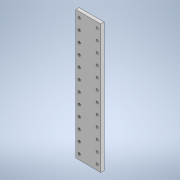
# Autodesk Inventor part: Base_plate
Saved by Autodesk Inventor 2022 (Build 260153000, 153)
## iProperties
Created: 2022-01-26
Part Number: Base_plate
Material: Generic
Document SubType Name: Modeling
Designer: Emazuddin Alif
Density: 1 g/cm^3
Appearance: Default
Author: Emazuddin Alif
Autodesk Inventor part; units mm, degrees
ref_plane "YZ Plane" through (0, 0, 0) normal (1, 0, 0) x (0, 1, 0)
ref_plane "XZ Plane" through (0, 0, 0) normal (0, 1, 0) x (-1, 0, 0)
ref_plane "XY Plane" through (0, 0, 0) normal (0, 0, 1) x (1, 0, 0)
sketch "Sketch1" plane through (0, 0, 0) normal (0, 0, 1) x (1, 0, 0)
  line L0 (44.45, -228.6) -> (-44.45, -228.6)
  line L1 (-44.45, -228.6) -> (-44.45, 228.6)
  line L2 (-44.45, 228.6) -> (44.45, 228.6)
  line L3 (44.45, 228.6) -> (44.45, -228.6)
  line L4 (44.45, -228.6) -> (-44.45, 228.6) construction
  line L5 (-44.45, -228.6) -> (44.45, 228.6) construction
  line L6 (0, 60.7039) -> (0, -84.4127)
  circle A0 centre (-31.75, -209.55) radius 3.9688
  circle A1 centre (31.75, -209.55) radius 3.9688
  circle A2 centre (-31.75, -171.45) radius 3.9688
  circle A3 centre (31.75, -171.45) radius 3.9688
  circle A4 centre (-31.75, -133.35) radius 3.9688
  circle A5 centre (31.75, -133.35) radius 3.9688
  circle A6 centre (-31.75, -95.25) radius 3.9688
  circle A7 centre (31.75, -95.25) radius 3.9688
  circle A8 centre (-31.75, -57.15) radius 3.9688
  circle A9 centre (31.75, -57.15) radius 3.9688
  circle A10 centre (-31.75, -19.05) radius 3.9688
  circle A11 centre (31.75, -19.05) radius 3.9688
  circle A12 centre (-31.75, 19.05) radius 3.9688
  circle A13 centre (31.75, 19.05) radius 3.9688
  circle A14 centre (-31.75, 57.15) radius 3.9688
  circle A15 centre (31.75, 57.15) radius 3.9688
  circle A16 centre (-31.75, 95.25) radius 3.9688
  circle A17 centre (31.75, 95.25) radius 3.9688
  circle A18 centre (-31.75, 133.35) radius 3.9688
  circle A19 centre (31.75, 133.35) radius 3.9688
  circle A20 centre (-31.75, 171.45) radius 3.9688
  circle A21 centre (31.75, 171.45) radius 3.9688
  circle A22 centre (-31.75, 209.55) radius 3.9688
  circle A23 centre (31.75, 209.55) radius 3.9688
  point P0 (0, 0)
  dimension "d0" = 457.2
  dimension "d1" = 88.9
  dimension "d2" = 7.9375
  dimension "d3" = 19.05
  dimension "d4" = 12.7
  dimension "d5" = 12.7
  dimension "d8" = 38.1
  constraints: 24 centre point, 14 end point, 2 midpoint, 2 parallel, 2 vertical, 1 horizontal, 1 perpendicular, 1 symmetric about line, 45 other
  measures "d0" distance of L0.end L1.end
  measures "d1" distance of L1.end L2.end
  measures "d2" diameter of A0
  measures "d3" distance from line of L0 A0.centre
  measures "d4" distance from line of L1 A0.centre
  measures "d5" distance from line of L3 A1.centre
  measures "d8" distance of A0.centre A2.centre
extrude "Extrusion1" add sketch "Sketch1" along normal blind 12.192
thread "Thread13" size "5/16-18 UNC" class "2B" standard "ANSI Unified Screw Threads" full length
thread "Thread14" size "5/16-18 UNC" class "2B" standard "ANSI Unified Screw Threads" full length
thread "Thread15" size "5/16-18 UNC" class "2B" standard "ANSI Unified Screw Threads" full length
thread "Thread16" size "5/16-18 UNC" class "2B" standard "ANSI Unified Screw Threads" full length
thread "Thread17" size "5/16-18 UNC" class "2B" standard "ANSI Unified Screw Threads" full length
thread "Thread18" size "5/16-18 UNC" class "2B" standard "ANSI Unified Screw Threads" full length
thread "Thread19" size "5/16-18 UNC" class "2B" standard "ANSI Unified Screw Threads" full length
thread "Thread20" size "5/16-18 UNC" class "2B" standard "ANSI Unified Screw Threads" full length
thread "Thread21" size "5/16-18 UNC" class "2B" standard "ANSI Unified Screw Threads" full length
thread "Thread22" size "5/16-18 UNC" class "2B" standard "ANSI Unified Screw Threads" full length
thread "Thread23" size "5/16-18 UNC" class "2B" standard "ANSI Unified Screw Threads" full length
thread "Thread24" size "5/16-18 UNC" class "2B" standard "ANSI Unified Screw Threads" full length
thread "Thread25" size "5/16-18 UNC" class "2B" standard "ANSI Unified Screw Threads" full length
thread "Thread26" size "5/16-18 UNC" class "2B" standard "ANSI Unified Screw Threads" full length
thread "Thread27" size "5/16-18 UNC" class "2B" standard "ANSI Unified Screw Threads" full length
thread "Thread28" size "5/16-18 UNC" class "2B" standard "ANSI Unified Screw Threads" full length
thread "Thread29" size "5/16-18 UNC" class "2B" standard "ANSI Unified Screw Threads" full length
thread "Thread30" size "5/16-18 UNC" class "2B" standard "ANSI Unified Screw Threads" full length
thread "Thread31" size "5/16-18 UNC" class "2B" standard "ANSI Unified Screw Threads" full length
thread "Thread32" size "5/16-18 UNC" class "2B" standard "ANSI Unified Screw Threads" full length
thread "Thread33" size "5/16-18 UNC" class "2B" standard "ANSI Unified Screw Threads" full length
thread "Thread34" size "5/16-18 UNC" class "2B" standard "ANSI Unified Screw Threads" full length
thread "Thread35" size "5/16-18 UNC" class "2B" standard "ANSI Unified Screw Threads" full length
thread "Thread36" size "5/16-18 UNC" class "2B" standard "ANSI Unified Screw Threads" full length
body "Solid1"
